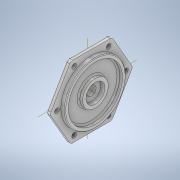
# Autodesk Inventor part: crank case cover
Saved by Autodesk Inventor 2021.1 (Build 251245000, 245)
## iProperties
Created: 2020-08-29
Part Number: crank case cover
Material: Aluminum 6061
Document SubType Name: Sheet Metal
Designer: Vamshi
Density: 2.7 g/cm^3
Sheet Metal Rule: Default
Appearance: Aluminum - Polished
Mass: 3254.8 g
Surface Area: 1682.39 cm^2
Volume: 1205.48 cm^3
Author: Vamshi
Autodesk Inventor part; units mm, degrees
ref_plane "YZ Plane" through (0, 0, 0) normal (1, 0, 0) x (0, 1, 0)
ref_plane "XZ Plane" through (0, 0, 0) normal (0, 1, 0) x (-1, 0, 0)
ref_plane "XY Plane" through (0, 0, 0) normal (0, 0, 1) x (1, 0, 0)
sketch "Sketch1" plane through (0, 0, 0) normal (0, 0, 1) x (1, 0, 0)
  line L0 (70.3905, -134.62) -> (-70.3905, -134.62)
  line L1 (-81.3891, -128.27) -> (-151.7796, -6.35)
  line L2 (-151.7796, 6.35) -> (-81.3891, 128.27)
  line L3 (-70.3905, 134.62) -> (70.3905, 134.62)
  line L4 (81.3891, 128.27) -> (151.7796, 6.35)
  line L5 (151.7796, -6.35) -> (81.3891, -128.27)
  arc A0 (-70.3905, 134.62) -> (-81.3891, 128.27) centre (-70.3905, 121.92) ccw
  arc A1 (-151.7796, 6.35) -> (-151.7796, -6.35) centre (-140.7811, 0) ccw
  arc A2 (-81.3891, -128.27) -> (-70.3905, -134.62) centre (-70.3905, -121.92) ccw
  arc A3 (70.3905, -134.62) -> (81.3891, -128.27) centre (70.3905, -121.92) ccw
  arc A4 (151.7796, -6.35) -> (151.7796, 6.35) centre (140.7811, 0) ccw
  arc A5 (81.3891, 128.27) -> (70.3905, 134.62) centre (70.3905, 121.92) ccw
  point P0 (0, 0)
  point P1 (0, 0)
  point P2 (77.7229, -134.62)
  point P3 (-77.7229, -134.62)
  point P4 (-155.4458, 0)
  point P5 (-77.7229, 134.62)
  point P6 (77.7229, 134.62)
  point P7 (155.4458, 0)
  dimension "d0" = 269.24
  dimension "d1" = 12.7
  constraints: 12 end point, 12 point on circle, 12 point on line, 12 tangent, 6 centre point, 5 equal radius, 1 coincident, 1 horizontal, 13 other
  measures "d0" distance between parallel lines of L0 L3
  measures "d1" radius of A0
extrude "Extrusion1" add sketch "Sketch1" along normal blind 15.24
sketch "Sketch2" plane through (0, 0, 15.24) normal (0, 0, 1) x (1, 0, 0)
  circle A0 centre (0, 0) radius 17.78
  circle A1 centre (0, 0) radius 58.42
  dimension "d5" = 35.56
  dimension "d8" = 116.84
  constraints: 2 centre point, 1 coincident
  measures "d5" diameter of A0
  measures "d8" diameter of A1
extrude "Extrusion2" cut sketch "Sketch2" against normal through all contours A0
sketch "Sketch3" plane through (0, 0, 0) normal (0, 0, -1) x (-1, 0, 0)
  circle A0 centre (0, 0) radius 17.78 projected
  circle A1 centre (0, 0) radius 58.42
  dimension "d9" = 116.84
  constraints: 1 centre point, 1 coincident
  measures "d9" diameter of A1
extrude "Extrusion3" add sketch "Sketch3" along normal blind 10.16
fillet "Fillet1" radius 10.16 1 edges at (58.42, 0, 0)
fillet "Fillet2" radius 5.08 12 edges at (-76.7405, 132.9185, 0) (-116.5843, 67.31, 0) (-153.4811, 0, 0) (-116.5843, -67.31, 0) (-76.7405, -132.9185, 0) (0, -134.62, 0) (76.7405, -132.9185, 0) (116.5843, -67.31, 0) (153.4811, 0, 0) (116.5843, 67.31, 0) (76.7405, 132.9185, 0) (0, 134.62, 0)
sketch "Sketch4" plane through (0, 0, 15.24) normal (0, 0, 1) x (1, 0, 0)
  circle A0 centre (0, 0) radius 129.54 construction
  circle A1 centre (0, 0) radius 35.56
  circle A2 centre (0, 0) radius 48.26
  circle A3 centre (0, 0) radius 17.78 projected
  circle A4 centre (0, 0) radius 101.6
  circle A5 centre (0, 0) radius 114.3
  circle A6 centre (-129.54, 0) radius 8.89
  circle A7 centre (-64.77, -112.1849) radius 8.89
  circle A8 centre (64.77, -112.1849) radius 8.89
  circle A9 centre (129.54, 0) radius 8.89
  circle A10 centre (64.77, 112.1849) radius 8.89
  circle A11 centre (-64.77, 112.1849) radius 8.89
  dimension "d14" = 259.08
  dimension "d15" = 71.12
  dimension "d16" = 96.52
  dimension "d17" = 203.2
  dimension "d18" = 228.6
  dimension "d19" = 17.78
  dimension "d22" = 360
  constraints: 10 centre point, 5 coincident, 1 horizontal alignment, 15 other
  measures "d15" diameter of A1
  measures "d16" diameter of A2
  measures "d17" diameter of A4
  measures "d18" diameter of A5
  measures "d19" diameter of A6
extrude "Extrusion4" add sketch "Sketch4" along normal blind 15.24 contours A2 | A5
extrude "Extrusion5" cut sketch "Sketch4" against normal through all contours A6 | A7 | A8 | A9 | A10 | A11
fillet "Fillet3" radius 5.08 2 edges at (-101.6, 0, 15.24) (-48.26, 0, 15.24)
chamfer "Chamfer1" distance 2.54 angle 45 1 edges at (-114.3, 0, 30.48)
equation "\"BendRadius\" = Thickness"
equation "\"BendReliefWidth\" = Thickness"
equation "\"BendReliefDepth\" = 0.5 * Thickness"
equation "\"CornerReliefSize\" = 4 * Thickness"
equation "\"MinimumRemnant\" = 2 * Thickness"
equation "\"TransitionRadius\" = BendRadius"
equation "\"JacobiRadiusSize\" = BendRadius"
equation "\"GapSize\" = Thickness"
equation "\"Thickness\" = 3.048"
body "Solid1"
